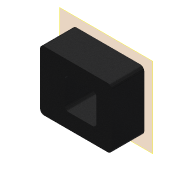
# Autodesk Inventor part: 00_Axiovert_focusblock
Saved by Autodesk Inventor 2019.4 (Build 234330000, 330)
## iProperties
Created: 2020-10-09
Part Number: 00_Axiovert_focusblock
Material: Generic
Document SubType Name: Modeling
Designer: diederichbenedict
Density: 1 g/cm^3
Appearance: Black Cast
Author: diederichbenedict
Autodesk Inventor part; units mm, degrees
note: some values were not read from the file. Chosen so that the rebuilt part matches the saved one: sketch regions of "Extrusion2".
ref_plane "YZ Plane" through (0, 0, 0) normal (1, 0, 0) x (0, 1, 0)
ref_plane "XZ Plane" through (0, 0, 0) normal (0, 1, 0) x (-1, 0, 0)
ref_plane "XY Plane" through (0, 0, 0) normal (0, 0, 1) x (1, 0, 0)
ref_plane "Work Plane1" through (0, 0, 0) normal (0, 0, 1) x (1, 0, 0)
sketch "Sketch1" plane through (0, 0, 0) normal (0, 0, 1) x (1, 0, 0)
  line L0 (-199.8571, 167.3322) -> (-0.3512, 153.2823) projected
  line L1 (-199.8571, 167.3322) -> (-212.6962, -14.9789) projected
  line L2 (-204.4935, -14.4012) -> (-212.6962, -14.9789) projected
  arc A0 (-204.4935, -14.4012) -> (-199.8571, -9.0623) centre (-204.8448, -9.4136) ccw projected
  line L3 (-0.3512, 4.9876) -> (-199.8571, -9.0623) projected
  line L4 (-0.3512, 4.9876) -> (-5.573, 79.1349) projected
  line L5 (-0.3512, 153.2823) -> (-5.573, 79.1349) projected
  line L6 (-21.5243, 154.0691) -> (-180.8464, 154.0691)
  line L7 (-190.8464, 144.0691) -> (-190.8464, 14.2008)
  line L8 (-180.8464, 4.2008) -> (-21.5243, 4.2008)
  line L9 (-11.5243, 14.2008) -> (-11.5243, 144.0691)
  circle A1 centre (-89.3933, 80.4886) radius 30.8095 projected
  line L10 (-59.7137, 118.9158) -> (-119.0729, 118.9158)
  line L11 (-129.0729, 108.9158) -> (-129.0729, 52.0613)
  line L12 (-119.0729, 42.0613) -> (-59.7137, 42.0613)
  line L13 (-49.7137, 52.0613) -> (-49.7137, 108.9158)
  line L14 (-49.7137, 118.9158) -> (-129.0729, 42.0613) construction
  line L15 (-129.0729, 118.9158) -> (-49.7137, 42.0613) construction
  arc A2 (-49.7137, 108.9158) -> (-59.7137, 118.9158) centre (-59.7137, 108.9158) ccw
  arc A3 (-59.7137, 42.0613) -> (-49.7137, 52.0613) centre (-59.7137, 52.0613) ccw
  arc A4 (-129.0729, 52.0613) -> (-119.0729, 42.0613) centre (-119.0729, 52.0613) ccw
  arc A5 (-119.0729, 118.9158) -> (-129.0729, 108.9158) centre (-119.0729, 108.9158) ccw
  arc A6 (-11.5243, 144.0691) -> (-21.5243, 154.0691) centre (-21.5243, 144.0691) ccw
  arc A7 (-21.5243, 4.2008) -> (-11.5243, 14.2008) centre (-21.5243, 14.2008) ccw
  arc A8 (-190.8464, 14.2008) -> (-180.8464, 4.2008) centre (-180.8464, 14.2008) ccw
  arc A9 (-180.8464, 154.0691) -> (-190.8464, 144.0691) centre (-180.8464, 144.0691) ccw
  point P0 (0, 0)
  point P1 (-11.5243, 154.0691)
  point P2 (-11.5243, 4.2008)
  dimension "d0" = 10
  constraints: 20 end point, 16 point on circle, 16 tangent, 14 point on line, 8 centre point, 7 equal radius, 4 parallel, 2 horizontal, 2 midpoint, 2 perpendicular
  measures "d0" radius of A2
extrude "Extrusion1" add sketch "Sketch1" along normal up to surface (81.1444 mm away) contours A6 L9 A7 L8 A8 L7 A9 L6
sketch "Sketch2" plane through (-180.8464, 154.0691, 81.1444) normal (0, 0, 1) x (1, 0, 0)
  arc A0 (121.1327, -112.0078) -> (131.1327, -102.0078) centre (121.1327, -102.0078) ccw projected
  line L0 (61.7735, -112.0078) -> (121.1327, -112.0078) projected
  arc A1 (51.7735, -102.0078) -> (61.7735, -112.0078) centre (61.7735, -102.0078) ccw projected
  line L1 (51.7735, -45.1533) -> (51.7735, -102.0078) projected
  arc A2 (61.7735, -35.1533) -> (51.7735, -45.1533) centre (61.7735, -45.1533) ccw projected
  line L2 (121.1327, -35.1533) -> (61.7735, -35.1533) projected
  arc A3 (131.1327, -45.1533) -> (121.1327, -35.1533) centre (121.1327, -45.1533) ccw projected
  line L3 (131.1327, -102.0078) -> (131.1327, -45.1533) projected
  arc A4 (159.322, -149.8683) -> (169.322, -139.8683) centre (159.322, -139.8683) ccw projected
  line L4 (169.322, -10) -> (169.322, -139.8683) projected
  arc A5 (169.322, -10) -> (159.322, 0) centre (159.322, -10) ccw projected
  line L5 (0, 0) -> (159.322, 0) projected
  arc A6 (0, 0) -> (-10, -10) centre (0, -10) ccw projected
  line L6 (-10, -139.8683) -> (-10, -10) projected
  arc A7 (-10, -139.8683) -> (0, -149.8683) centre (0, -139.8683) ccw projected
  line L7 (159.322, -149.8683) -> (0, -149.8683) projected
  line L8 (23.5841, -179.6476) -> (159.322, -179.6476)
  line L9 (169.322, -169.6476) -> (169.322, 19.7793)
  line L10 (159.322, 29.7793) -> (23.5841, 29.7793)
  line L11 (13.5841, 19.7793) -> (13.5841, -169.6476)
  line L12 (13.5841, -179.6476) -> (169.322, 29.7793) construction
  line L13 (169.322, -179.6476) -> (13.5841, 29.7793) construction
  arc A8 (169.322, 19.7793) -> (159.322, 29.7793) centre (159.322, 19.7793) ccw
  arc A9 (23.5841, 29.7793) -> (13.5841, 19.7793) centre (23.5841, 19.7793) ccw
  arc A10 (13.5841, -169.6476) -> (23.5841, -179.6476) centre (23.5841, -169.6476) ccw
  arc A11 (159.322, -179.6476) -> (169.322, -169.6476) centre (159.322, -169.6476) ccw
  point P0 (180.8464, -154.0691)
  point P1 (91.4531, -74.9342)
  dimension "d3" = 10
  constraints: 12 end point, 8 point on circle, 8 point on line, 8 tangent, 4 centre point, 3 equal radius, 2 midpoint, 2 parallel, 1 horizontal, 1 perpendicular
  measures "d3" radius of A8
extrude "Extrusion2" add sketch "Sketch2" along normal blind 10
body "Solid1"
